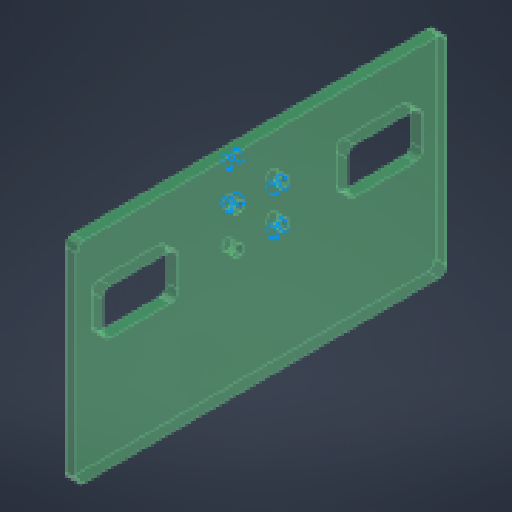
# Autodesk Inventor part: PARED FRONTAL
Saved by Autodesk Inventor 2026.2 (Build 302298010, 298A)
## iProperties
Created: 2026-02-05
Part Number: PARED FRONTAL
Material: Generic
Document SubType Name: Modeling
Designer: 06aar
Density: 1 g/cm^3
Appearance: Clear - Green 1
Author: 06aar
Autodesk Inventor part; units mm, degrees
ref_plane "YZ Plane" through (0, 0, 0) normal (1, 0, 0) x (0, 1, 0)
ref_plane "XZ Plane" through (0, 0, 0) normal (0, 1, 0) x (-1, 0, 0)
ref_plane "XY Plane" through (0, 0, 0) normal (0, 0, 1) x (1, 0, 0)
sketch "Sketch1" plane through (0, 0, 0) normal (1, 0, 0) x (0, 1, 0)
  line L0 (2, 0) -> (54, 0)
  line L1 (56, -2) -> (56, -96.5)
  line L2 (54, -98.5) -> (2, -98.5)
  line L3 (0, -96.5) -> (0, -2)
  line L4 (40, -7) -> (32, -7)
  line L5 (30, -9) -> (30, -25)
  line L6 (32, -27) -> (40, -27)
  line L7 (42, -25) -> (42, -9)
  arc A0 (40, -27) -> (42, -25) centre (40, -25) ccw
  arc A1 (32, -7) -> (30, -9) centre (32, -9) ccw
  arc A2 (30, -25) -> (32, -27) centre (32, -25) ccw
  arc A3 (42, -9) -> (40, -7) centre (40, -9) ccw
  line L8 (0, -49.5) -> (56, -49.5)
  line L9 (40, -92) -> (32, -92)
  line L10 (30, -90) -> (30, -74)
  line L11 (32, -72) -> (40, -72)
  line L12 (42, -74) -> (42, -90)
  arc A4 (42, -74) -> (40, -72) centre (40, -74) ccw
  arc A5 (30, -90) -> (32, -92) centre (32, -90) ccw
  arc A6 (32, -72) -> (30, -74) centre (32, -74) ccw
  arc A7 (40, -92) -> (42, -90) centre (40, -90) ccw
  arc A8 (56, -2) -> (54, 0) centre (54, -2) ccw
  arc A9 (54, -98.5) -> (56, -96.5) centre (54, -96.5) ccw
  arc A10 (0, -96.5) -> (2, -98.5) centre (2, -96.5) ccw
  arc A11 (2, 0) -> (0, -2) centre (2, -2) ccw
  point P0 (0, 0)
  point P1 (56, -98.5)
  point P2 (56, 0)
  point P3 (0, -98.5)
  point P4 (42, -7)
  point P5 (30, -27)
  point P6 (42, -27)
  point P7 (42, -92)
  point P8 (30, -72)
  point P9 (42, -72)
  dimension "d0" = 56
  dimension "d1" = 98.5
  dimension "d2" = 7
  dimension "d3" = 30
  dimension "d4" = 12
  dimension "d5" = 20
  dimension "d6" = 2
  dimension "d7" = 49.5
  dimension "d10" = 2
  constraints: 26 end point, 24 point on circle, 22 point on line, 16 tangent, 15 symmetric about line, 12 centre point, 6 equal radius, 4 parallel, 3 perpendicular, 2 horizontal, 4 other
  measures "d0" distance of point (56, -98.5) point (0, -98.5)
  measures "d1" distance of point (0, -98.5) point (0, 0)
  measures "d2" distance between parallel lines of L0 L4
  measures "d3" distance between parallel lines of L5 L3
  measures "d4" distance of point (30, -27) point (42, -27)
  measures "d5" distance of point (42, -27) point (42, -7)
  measures "d6" radius of A0
  measures "d7" distance between parallel lines of L0 L8
  measures "d10" radius of A8
extrude "Extrusion1" add sketch "Sketch1" along normal blind 3
sketch "Boceto2" plane through (3, 0, 0) normal (1, 0, 0) x (0, 0, -1)
  circle A0 centre (43.0768, 43) radius 1.5 construction
  circle A1 centre (55.0768, 43) radius 1.5 construction
  circle A2 centre (43.0768, 33) radius 1.5 construction
  circle A3 centre (55.0768, 33) radius 1.5 construction
  point P0 (0, 0)
hole "SpacersSetHerramientas" at (3, 43, -43.0768) at (3, 33, -43.0768) at (3, 33, -55.0768) at (3, 43, -55.0768) direction (-1, 0, 0) diameter 3 end through all
body "Solid1"
